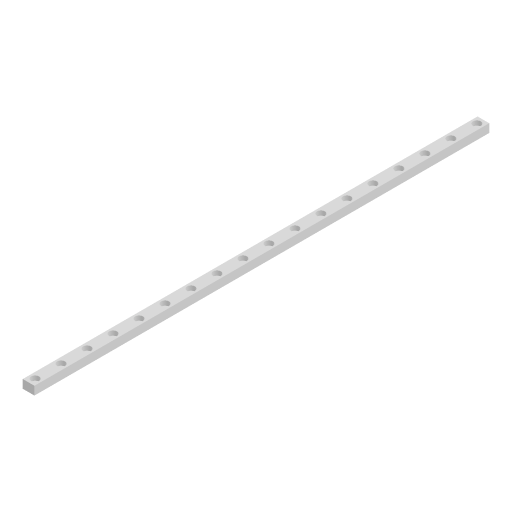
# Autodesk Inventor part: mgn9 350mm
Saved by Autodesk Inventor 2023 (Build 270158000, 158)
## iProperties
Created: 2022-09-16
Part Number: mgn9 350mm
Material: Generic
Document SubType Name: Modeling
Designer: deli
Density: 1 g/cm^3
Appearance: Default
Author: deli
Autodesk Inventor part; units mm, degrees
ref_plane "YZ Plane" through (0, 0, 0) normal (1, 0, 0) x (0, 1, 0)
ref_plane "XZ Plane" through (0, 0, 0) normal (0, 1, 0) x (-1, 0, 0)
ref_plane "XY Plane" through (0, 0, 0) normal (0, 0, 1) x (1, 0, 0)
sketch "Sketch4" plane through (0, 0, 0) normal (0, 0, 1) x (1, 0, 0)
  line L0 (-22.685, 6.9816) -> (-13.685, 6.9816)
  line L1 (-13.685, 6.9816) -> (-13.685, 0.4816)
  line L2 (-13.685, 0.4816) -> (-22.685, 0.4816)
  line L3 (-22.685, 0.4816) -> (-22.685, 6.9816)
  point P0 (0, 0)
  dimension "d27" = 9
  dimension "d28" = 6.5
  constraints: 8 end point, 2 parallel, 1 horizontal, 1 perpendicular
  measures "d27" distance of L1.end L2.end
  measures "d28" distance of L0.end L1.end
extrude "Extrusion3" add sketch "Sketch4" along normal blind 350
sketch "Sketch9" plane through (-22.685, 6.9816, 0) normal (0, 1, 0) x (1, 0, 0)
  circle A0 centre (4.5, -345) radius 1.75
  line L0 (0, 0) -> (0, -350) projected
  circle A1 centre (4.5, -325) radius 1.75
  circle A2 centre (4.5, -305) radius 1.75
  circle A3 centre (4.5, -285) radius 1.75
  circle A4 centre (4.5, -265) radius 1.75
  circle A5 centre (4.5, -245) radius 1.75
  circle A6 centre (4.5, -225) radius 1.75
  circle A7 centre (4.5, -205) radius 1.75
  circle A8 centre (4.5, -185) radius 1.75
  circle A9 centre (4.5, -165) radius 1.75
  circle A10 centre (4.5, -145) radius 1.75
  circle A11 centre (4.5, -125) radius 1.75
  circle A12 centre (4.5, -105) radius 1.75
  circle A13 centre (4.5, -85) radius 1.75
  circle A14 centre (4.5, -65) radius 1.75
  circle A15 centre (4.5, -45) radius 1.75
  circle A16 centre (4.5, -25) radius 1.75
  circle A17 centre (4.5, -5) radius 1.75
  line L1 (9, -350) -> (0, -350) projected
  point P0 (22.685, 0)
  dimension "d61" = 3.5
  dimension "d62" = 4.5
  dimension "d68" = 20
  dimension "d70" = 340
  dimension "d71" = 5
  constraints: 18 centre point, 1 vertical, 34 other
  measures "d61" diameter of A0
  measures "d62" distance from line of L0 A0.centre
  measures "d68" distance of A0.centre A1.centre
  measures "d70" distance of A17.centre A0.centre
  measures "d71" distance from line of L1 A0.centre
extrude "Extrusion8" cut sketch "Sketch9" against normal blind 10
sketch "Sketch10" plane through (-22.685, 6.9816, 0) normal (0, 1, 0) x (1, 0, 0)
  circle A0 centre (4.5, -345) radius 1.75 construction
  circle A1 centre (4.5, -345) radius 3
  line L0 (0, 0) -> (0, -350) projected
  circle A2 centre (4.5, -325) radius 3
  circle A3 centre (4.5, -305) radius 3
  circle A4 centre (4.5, -285) radius 3
  circle A5 centre (4.5, -265) radius 3
  circle A6 centre (4.5, -245) radius 3
  circle A7 centre (4.5, -225) radius 3
  circle A8 centre (4.5, -205) radius 3
  circle A9 centre (4.5, -185) radius 3
  circle A10 centre (4.5, -165) radius 3
  circle A11 centre (4.5, -145) radius 3
  circle A12 centre (4.5, -125) radius 3
  circle A13 centre (4.5, -105) radius 3
  circle A14 centre (4.5, -85) radius 3
  circle A15 centre (4.5, -65) radius 3
  circle A16 centre (4.5, -45) radius 3
  circle A17 centre (4.5, -25) radius 3
  circle A18 centre (4.5, -5) radius 3
  point P0 (22.685, 0)
  dimension "d74" = 6
  dimension "d80" = 20
  constraints: 18 centre point, 1 coincident, 1 vertical, 34 other
  measures "d74" diameter of A1
  measures "d80" distance of A1.centre A2.centre
extrude "Extrusion9" cut sketch "Sketch10" against normal blind 3.5
body "Solid2"
